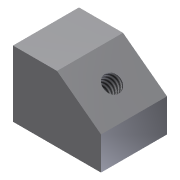
# Autodesk Inventor part: transfer mount block
Saved by Autodesk Inventor 2012 (Build 160160000, 160)
## iProperties
Created: 2012-04-25
Part Number: transfer mount block
Material: Default
Document SubType Name: Modeling
Designer: Antonella Wilby
Density: 1 g/cm^3
Author: Antonella Wilby
Autodesk Inventor part; units mm, degrees
ref_plane "YZ Plane" through (0, 0, 0) normal (1, 0, 0) x (0, 1, 0)
ref_plane "XZ Plane" through (0, 0, 0) normal (0, 1, 0) x (-1, 0, 0)
ref_plane "XY Plane" through (0, 0, 0) normal (0, 0, 1) x (1, 0, 0)
sketch "Sketch1" plane through (0, 0, 0) normal (0, 0, 1) x (1, 0, 0)
  line L0 (-23.0956, 0) -> (12.4644, 0) projected
  line L1 (0, -13.335) -> (0, 13.335) projected
  line L2 (-18.0156, 9.525) -> (-5.3156, 9.525)
  line L3 (7.3844, 0) -> (7.3844, -9.525)
  line L4 (7.3844, -9.525) -> (-18.0156, -9.525)
  line L5 (-18.0156, -9.525) -> (-18.0156, 9.525)
  line L6 (-5.3156, 9.525) -> (7.3844, 0)
  point P0 (0, 0)
  point P1 (-18.0156, 0)
  point P2 (0, 9.525)
  dimension "d0" = 19.05
  dimension "d1" = 12.7
  dimension "d2" = 25.4
  constraints: 10 end point, 2 parallel, 1 horizontal, 1 horizontal alignment, 1 midpoint, 1 perpendicular, 1 vertical alignment
  measures "d0" distance of L4.end L2.start
  measures "d1" distance of L2.start L2.end
  measures "d2" distance of L3.end L4.end
extrude "Extrusion1" add sketch "Sketch1" along normal blind 19.05
sketch "Sketch2" plane through (7.3844, 0, 19.05) normal (0.6, 0.8, 0) x (0.8, -0.6, 0)
  line L0 (-15.875, 19.05) -> (0, 19.05) projected
  line L1 (-15.875, 19.05) -> (-15.875, 0) projected
  point P0 (-5.9075, 19.05)
  point P1 (-7.9375, 9.525)
  point P2 (-15.875, 9.525)
  point P3 (-7.9375, 19.05)
  constraints: 2 midpoint, 1 horizontal alignment, 1 vertical alignment
hole "Hole1" at (1.0344, 4.7625, 9.525) direction (-0.6, -0.8, 0) diameter 4.9784 end through all thread size "1/4-20 UNC" class "2B" standard "ANSI Unified Screw Threads"
sketch "Sketch3" plane through (-18.0156, -9.525, 0) normal (0, -1, 0) x (1, 0, 0)
  line L0 (25.4, 0) -> (25.4, 19.05) projected
  point P0 (18.0156, 0)
  point P1 (19.05, 9.525)
  point P2 (25.4, 9.525)
  point P3 (3.175, 9.525)
  dimension "d12" = 6.35
  dimension "d20" = 15.875
  constraints: 2 horizontal alignment, 1 midpoint
  measures "d12" distance from line of L0 point (19.05, 9.525)
  measures "d20" distance of point (19.05, 9.525) point (3.175, 9.525)
hole "Hole2" at (1.0344, -9.525, 9.525) at (-14.8406, -9.525, 9.525) direction (0, 1, 0) diameter 4.9784 depth 6.35 tip angle 118 thread size "1/4-20 UNC" class "2B" standard "ANSI Unified Screw Threads"
body "Solid1"
